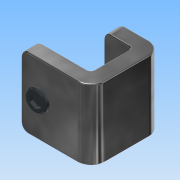
# Autodesk Inventor part: скоба
Saved by Autodesk Inventor 2017 (Build 210142000, 142)
## iProperties
Part Number: скоба
Material: Типовые
Document SubType Name: Modeling
Designer: Max
Mass: 0.448147 g
Surface Area: 5.37256 cm^2
Volume: 0.448147 cm^3
Density: 1 g/cm^3
Appearance: Сталь - гальванизированная
Author: Max
Autodesk Inventor part; units mm, degrees
ref_plane "YZ Plane" through (0, 0, 0) normal (1, 0, 0) x (0, 1, 0)
ref_plane "XZ Plane" through (0, 0, 0) normal (0, 1, 0) x (-1, 0, 0)
ref_plane "XY Plane" through (0, 0, 0) normal (0, 0, 1) x (1, 0, 0)
sketch "Эскиз1" plane through (0, 0, 0) normal (0, 0, 1) x (1, 0, 0)
  line L0 (-2, 0) -> (-9.9, 0)
  line L1 (-6.2, 10) -> (-2, 10)
  line L2 (0, 8) -> (0, 2)
  line L3 (-6.2, 7.9) -> (-2.7, 7.9)
  line L4 (-2.2, 7.4) -> (-2.2, 2.6)
  line L5 (-2.7, 2.1) -> (-9.9, 2.1)
  line L6 (0, 5) -> (-10, 5) construction
  line L7 (-6.2, 10) -> (-6.2, 7.9)
  line L8 (-9.9, 0) -> (-9.9, 2.1)
  arc A0 (0, 8) -> (-2, 10) centre (-2, 8) ccw
  arc A1 (-2, 0) -> (0, 2) centre (-2, 2) ccw
  arc A2 (-2.2, 7.4) -> (-2.7, 7.9) centre (-2.7, 7.4) ccw
  arc A3 (-2.7, 2.1) -> (-2.2, 2.6) centre (-2.7, 2.6) ccw
  point P0 (0, 0)
  dimension "d0" = 10
  dimension "d1" = 5.8
  dimension "d2" = 2.1
  dimension "d3" = 2.2
  dimension "d5" = 6.2
  dimension "d6" = 9.9
  dimension "d7" = 2
  dimension "d8" = 2.1
  dimension "d9" = 0.5
  constraints: 18 end point, 8 point on circle, 8 tangent, 4 centre point, 4 perpendicular, 3 parallel, 2 equal radius, 2 horizontal, 2 point on line, 1 midpoint, 1 other
  measures "d0" distance between parallel lines of L0 L1
  measures "d1" distance between parallel lines of L3 L5
  measures "d2" distance between parallel lines of L1 L3
  measures "d3" distance between parallel lines of L2 L4
  measures "d5" distance between parallel lines of L2 L7
  measures "d6" distance between parallel lines of L2 L8
  measures "d7" radius of A0
  measures "d8" distance between parallel lines of L0 L5
  measures "d9" radius of A2
extrude "Выдавливание1" add sketch "Эскиз1" along normal mid plane 9.9
fillet "Сопряжение1" radius 1 4 edges at (-6.2, 8.95, 4.95) (-6.2, 8.95, -4.95) (-9.9, 1.05, 4.95) (-9.9, 1.05, -4.95)
fillet "Сопряжение2" radius 0.2 32 edges at (-9.6071, 2.1, 4.6571) (-9.9, 2.1, 0) (-9.6071, 2.1, -4.6571) (-5.8, 2.1, -4.95) (-2.3464, 2.2464, -4.95) (-2.2, 5, -4.95) (-2.3464, 7.7536, -4.95) (-3.95, 7.9, -4.95) (-5.9071, 7.9, -4.6571) (-6.2, 7.9, 0) (-5.9071, 7.9, 4.6571) (-3.95, 7.9, 4.95) (-2.3464, 7.7536, 4.95) (-2.2, 5, 4.95) (-2.3464, 2.2464, 4.95) (-5.8, 2.1, 4.95) (-0.5858, 0.5858, 4.95) (0, 5, 4.95) (-0.5858, 9.4142, 4.95) (-3.6, 10, 4.95) (-5.9071, 10, 4.6571) (-6.2, 10, 0) (-5.9071, 10, -4.6571) (-3.6, 10, -4.95) (-0.5858, 9.4142, -4.95) (0, 5, -4.95) (-0.5858, 0.5858, -4.95) (-5.45, 0, -4.95) (-9.6071, 0, -4.6571) (-9.9, 0, 0) (-9.6071, 0, 4.6571) (-5.45, 0, 4.95)
sketch "Эскиз2" plane through (-8.9, 0, -4.75) normal (0, -1, 0) x (1, 0, 0)
  line L0 (-1, 8.7) -> (-1, 0.8) construction
  line L1 (-1, 4.75) -> (9.4252, 4.75) construction
  circle A0 centre (1.5, 4.75) radius 1.5
  point P0 (8.9, 4.75)
  dimension "d14" = 3
  dimension "d15" = 2.5
  constraints: 2 end point, 1 centre point, 1 horizontal, 1 midpoint, 1 point on line
  measures "d14" diameter of A0
  measures "d15" distance from line of L0 A0.centre
extrude "Выдавливание2" add sketch "Эскиз2" against normal blind 2.6 and the other way blind 0.5
chamfer "Фаска1" distance 0.2 angle 45 1 edges at (-8.9, -0.5, 0)
sketch "Эскиз3" plane through (-7.4, -0.5, 0) normal (0, -1, 0) x (1, 0, 0)
  line L0 (0.004, 0.8904) -> (0.7731, 0.4417)
  line L1 (0.7731, 0.4417) -> (0.7691, -0.4487)
  line L2 (0.7691, -0.4487) -> (-0.004, -0.8904)
  line L3 (-0.004, -0.8904) -> (-0.7731, -0.4417)
  line L4 (-0.7731, -0.4417) -> (-0.7691, 0.4487)
  line L5 (-0.7691, 0.4487) -> (0.004, 0.8904)
  point P0 (7.4, 0)
  point P1 (0, 0)
  constraints: 12 end point, 13 other
extrude "Выдавливание3" cut sketch "Эскиз3" against normal blind 0.5
